Starting blocs_v2 (Autodesk Fusion 360 design; units mm, degrees)
Autodesk Fusion 360 part; units mm, degrees
sketch "Esquisse1" plane through (0, 0, 0) normal (0, 0, 1) x (1, 0, 0)
  line L0 (0, 0) -> (50, 0)
  line L1 (50, 0) -> (50, 37.5)
  line L2 (50, 37.5) -> (0, 37.5)
  line L3 (0, 37.5) -> (0, 0)
  dimension "d1" = 50
  dimension "d2" = 37.5
  constraint horizontal L0
  constraint vertical L1
  constraint horizontal L2
  constraint vertical L3
  constraint coincident L0.start L3.end
  measures "d1" distance of L0.start L0.end
  measures "d2" distance of L0.start L2.end
extrude "Extrusion1" add sketch "Esquisse1" along normal blind 50
fillet "Congé1" radius 1 5 faces at (16.6667, 25, 50) (0, 25, 16.6667) (16.6667, 0, 16.6667) (33.3333, 37.5, 16.6667) (50, 12.5, 16.6667)
equation "d2 = pipe_diameter + pipe_wall_distance"
equation "pipe_diameter = 34 mm"
equation "pipe_wall_distance = 3.5 mm"
